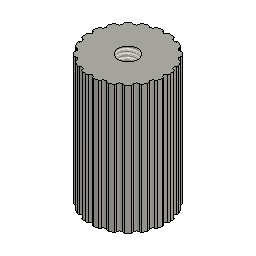
Claw (Autodesk Fusion 360 design; units mm, degrees)
part number: 2026-04-18-16-56-58-172
Autodesk Fusion 360 part; units mm, degrees
sketch "Sketch5" plane through (0, 0, 0) normal (0, 0, 1) x (1, 0, 0)
  circle A0 centre (0, 0) radius 7.5
  dimension "d23" = 15
  constraint coincident A0.centre origin
  measures "d23" diameter of A0
extrude "Extrude5" add sketch "Sketch5" along normal blind 25
sketch "Sketch6" plane through (0, 0, 25) normal (0, 0, 1) x (-1, 0, 0)
  circle A0 centre (0, 0) radius 7.5
  circle A1 centre (0, 0) radius 2.25
  dimension "d26" = 4.5
  constraint coincident A0.centre A1.centre
  measures "d26" diameter of A1
extrude "Extrude6" cut sketch "Sketch6" against normal blind 15 contours A1
thread "Thread3" "ISO Metric profile 4.5 M4.5x0.75 M4.5x0.75 6H" major diameter 4.6131 minor diameter 3.7831 pitch 0.75 angle 60 resizes the face on face at (-2.2388, 0.224, 15)
sketch "Sketch7" plane through (0, 0, 25) normal (0, 0, 1) x (-1, 0, 0)
  circle A0 centre (0, 0) radius 1.8916
  circle A1 centre (0, 0) radius 7.5
  circle A2 centre (7.5, 0) radius 0.5
  dimension "d31" = 1
  constraint coincident A1 A2.centre
  measures "d31" diameter of A2
extrude "Extrude7" cut sketch "Sketch7" against normal blind 25 contours A1 A2 picked at (7.3438, -0.1152)
fillet "Fillet1" radius 0.3 2 edges at (-7.4833, -0.4997, 12.5) (-7.4833, 0.4997, 12.5)
pattern_circular "C-Pattern2" count 20 over 360 about axis through (0, 0, 1.75) along (0, 0, 1) of "Extrude7", "Fillet1"
